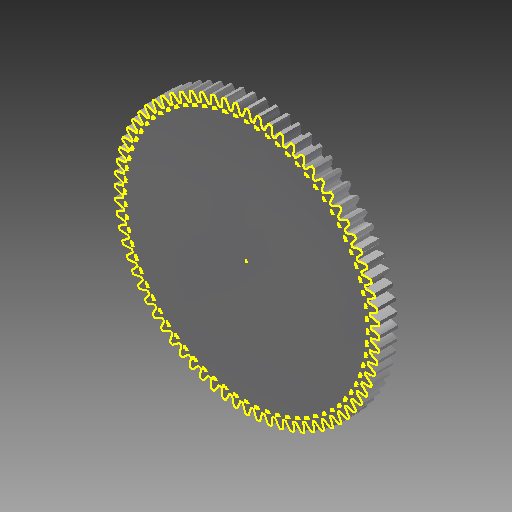
# Autodesk Inventor part: Цилиндрическое зубчатое зацепление2
Saved by Autodesk Inventor 2019 (Build 230136000, 136)
## iProperties
Created: 2020-02-27
Part Number: Цилиндрическое зубчатое зацепление2
Material: Steel
Document SubType Name: Modeling
Designer: Петров Иван
Categories: <?xml version="1.0" encoding="UTF-16"?> <MemberInstance><Categories><FamilyTemplate><FamilyTemplateParameter ValueType="xs:double" Id="1" ObjectReferenceKey="da_z" ObjectType="kUserParameterObject"/><FamilyTemplateParameter ValueType="xs:double" Id="2" ObjectReferenceKey="da_b" ObjectType="kUserParameterObject"/><FamilyTemplateParameter ValueType="xs:double" Id="3" ObjectReferenceKey="da_beta" ObjectType="kUserParameterObject"/><FamilyTemplateParameter ValueType="xs:double" Id="4" ObjectReferenceKey="da_da" ObjectType="kUserParameterObject"/><FamilyTemplateParameter ValueType="xs:double" Id="5" ObjectReferenceKey="da_aw" ObjectType="kUserParameterObject"/><FamilyTemplateParameter ValueType="xs:string" Id="6" ObjectReferenceKey="EAIAABAAAACIAQAAAAAAAIAAAAAAAAAA" ObjectType="83910656" SubObjectId="SurfaceGeometry"/></FamilyTemplate><ParamToTemplateMap><ParamToTemplate CategoryParameter="//CategoryParameter[@InternalName='046C89C9-8512-4d59-83FE-43B91F4F132A']" TemplateParameter="1"/><ParamToTemplate CategoryParameter="//CategoryParameter[@InternalName='2552DF32-E462-4b46-AEBF-C6C7768E72AC']" TemplateParameter="2"/><ParamToTemplate CategoryParameter="//CategoryParameter[@InternalName='C9EE641D-15FC-4fae-A226-E94C4372FDD7']" TemplateParameter="3"/><ParamToTemplate><ParamToTemplate CategoryParameter="//CategoryParameter[@InternalName='00B6519A-459B-49c7-AD84-2E56D39A5744']" ConstantValue="-1.297544"/></ParamToTemplate><ParamToTemplate><ParamToTemplate CategoryParameter="//CategoryParameter[@InternalName='04B31F0E-C7A6-4894-AA32-9629BEFACF47']" ConstantValue="1.000000"/></ParamToTemplate><ParamToTemplate><ParamToTemplate CategoryParameter="//CategoryParameter[@InternalName='43CBEC2E-7847-49e7-A936-2F7889FCB2D9']" ConstantValue="0.250000"/></ParamToTemplate><ParamToTemplate><ParamToTemplate CategoryParameter="//CategoryParameter[@InternalName='B1EFC894-105D-4ebd-86BF-FA20ED196853']" ConstantValue="0.350000"/></ParamToTemplate><ParamToTemplate><ParamToTemplate CategoryParameter="//CategoryParameter[@InternalName='51175063-3D10-4879-93E8-6246FE8B403D']" ConstantValue="2060000000.000000"/></ParamToTemplate><ParamToTemplate><ParamToTemplate CategoryParameter="//CategoryParameter[@InternalName='A3A52E27-4454-46a9-B0BD-C932399B70AF']" ConstantValue="0.300000"/></ParamToTemplate><ParamToTemplate><ParamToTemplate CategoryParameter="//CategoryParameter[@InternalName='91B76062-C214-41d9-B1B9-14D2AB99603D']" ConstantValue="0.137500"/></ParamToTemplate><ParamToTemplate><ParamToTemplate CategoryParameter="//CategoryParameter[@InternalName='374E806E-8B8A-4dda-A9AA-1039D6500AD2']" ConstantValue="7.272727"/></ParamToTemplate><ParamToTemplate><ParamToTemplate CategoryParameter="//CategoryParameter[@InternalName='2D373A89-B862-43d6-8D0B-0CBF12AB9F6C']" ConstantValue="0.523599"/></ParamToTemplate><ParamToTemplate CategoryParameter="//CategoryParameter[@InternalName='37777632-D6A2-4fac-9D53-DB8ACD95C989']" TemplateParameter="4"/><ParamToTemplate CategoryParameter="//CategoryParameter[@InternalName='FD1017F1-B727-4f7e-9707-0F86F1FF9423']" TemplateParameter="5"/><ParamToTemplate><ParamToTemplate CategoryParameter="//CategoryParameter[@InternalName='9E1B4470-B2D3-4ff1-B813-535BB4CDF51A']" ConstantValue="3520000.000000"/></ParamToTemplate><ParamToTemplate><ParamToTemplate CategoryParameter="//CategoryParameter[@InternalName='F8452263-BFF6-458c-9FB1-07C4B99E95CD']" ConstantValue="11400000.000000"/></ParamToTemplate><ParamToTemplate><ParamToTemplate CategoryParameter="//CategoryParameter[@InternalName='3E3BB259-FD49-497f-8171-6EBC954A3479']" ConstantValue="2.000000"/></ParamToTemplate><ParamToTemplate CategoryParameter="//CategoryParameter[@InternalName='27C3BAF2-7550-4e4b-AE2C-0DB134B7D9B7']" TemplateParameter="6"/></ParamToTemplateMap><Category DisplayName="Gear" InternalName="DC85795E-93AB-48d5-8EEE-5A27447B64BD" Mnemonic="Gear"><CategoryParameter DisplayName="z" InternalName="046C89C9-8512-4d59-83FE-43B91F4F132A" Mnemonic="z"/><CategoryParameter DisplayName="b" InternalName="2552DF32-E462-4b46-AEBF-C6C7768E72AC" Mnemonic="b"/><CategoryParameter DisplayName="||b|" InternalName="C9EE641D-15FC-4fae-A226-E94C4372FDD7" Mnemonic="beta"/><CategoryParameter DisplayName="x" InternalName="00B6519A-459B-49c7-AD84-2E56D39A5744" Mnemonic="x"/><CategoryParameter DisplayName="a*" InternalName="04B31F0E-C7A6-4894-AA32-9629BEFACF47" Mnemonic="a"/><CategoryParameter DisplayName="c*" InternalName="43CBEC2E-7847-49e7-A936-2F7889FCB2D9" Mnemonic="c"/><CategoryParameter DisplayName="r|.f|*" InternalName="B1EFC894-105D-4ebd-86BF-FA20ED196853" Mnemonic="rf"/><CategoryParameter DisplayName="E" InternalName="51175063-3D10-4879-93E8-6246FE8B403D" Mnemonic="E"/><CategoryParameter DisplayName="||m|" InternalName="A3A52E27-4454-46a9-B0BD-C932399B70AF" Mnemonic="mi"/><Category DisplayName="SpurGear" InternalName="26C5A22E-A91E-4dfd-A3B3-23CCAFAE1764" Mnemonic="SpurGear"><CategoryParameter DisplayName="m" InternalName="91B76062-C214-41d9-B1B9-14D2AB99603D" Mnemonic="m"/><CategoryParameter DisplayName="P" InternalName="374E806E-8B8A-4dda-A9AA-1039D6500AD2" Mnemonic="PP"/><CategoryParameter DisplayName="||a|" InternalName="2D373A89-B862-43d6-8D0B-0CBF12AB9F6C" Mnemonic="alpha"/><CategoryParameter DisplayName="d|.a|" InternalName="37777632-D6A2-4fac-9D53-DB8ACD95C989" Mnemonic="da"/><CategoryParameter DisplayName="a|.w|" InternalName="FD1017F1-B727-4f7e-9707-0F86F1FF9423" Mnemonic="aw"/><CategoryParameter DisplayName="||s||.Flim|" InternalName="9E1B4470-B2D3-4ff1-B813-535BB4CDF51A" Mnemonic="sFlim"/><CategoryParameter DisplayName="||s||.Hlim|" InternalName="F8452263-BFF6-458c-9FB1-07C4B99E95CD" Mnemonic="sHlim"/><CategoryParameter DisplayName="тип" InternalName="3E3BB259-FD49-497f-8171-6EBC954A3479" Mnemonic="type"/><CategoryParameter DisplayName="PitchDiameter" InternalName="27C3BAF2-7550-4e4b-AE2C-0DB134B7D9B7" Mnemonic="IDS_PITCHDIAM"/></Category></Category></Categories></MemberInstance>
Density: 1 g/cm^3
Appearance: Steel
CustomPartVersion: 1
Author: Петров Иван
Autodesk Inventor part; units mm, degrees
sketch "Sketch1" plane through (0, 0, 0) normal (0, 0, 1) x (1, 0, 0)
  circle A0 centre (0, 0) radius 49
  dimension "d0" = 98
  constraints: 1 centre point
  measures "d0" diameter of A0
extrude "Extrusion1" add sketch "Sketch1" along normal blind 7
ref_plane "Work Plane2" through (0, 0, 3.5) normal (0, 0, 1) x (1, 0, 0)
sketch "Sketch2" plane through (0, 0, 0) normal (0, 0, -1) x (-1, 0, 0)
  circle A0 centre (0, 0) radius 49 projected
  circle A1 centre (0, 0) radius 48
  dimension "d3" = 96
  constraints: 1 centre point, 1 coincident
  measures "d3" diameter of A1
surface extrude "Средний диаметр" sketch "Sketch2" against normal through all shown no curves A1
ref_plane "Work Plane8" through (0, 0, 0) normal (0.9990482, 0.0436194, 0) x (0, 0, 1)
ref_plane "Work Plane9" through (0, 0, 0) normal (1, 0, 0) x (0, 1, 0)
spur gear teeth "Цилиндрическое зубчатое зацепление" teeth 72 pitch diameter 99 tip diameter 98 root diameter 91.9943 face width 7 start plane through (0, 0, 0) normal (0, 0, -1) x (-1, 0, 0)
sketch "Эскиз3" plane through (0, 0, 7) normal (0, 0, 1) x (1, 0, 0)
  arc A0 (4.8028, -48.7641) -> (5.506, -45.6664) centre (-12.0114, -43.3185) ccw projected
  arc A1 (5.506, -45.6664) -> (6.5009, -45.5354) centre (0, 0) ccw projected
  arc A2 (6.5009, -45.5354) -> (7.9819, -48.3455) centre (22.8137, -38.7337) ccw projected
  arc A3 (7.9819, -48.3455) -> (9.0346, -48.1599) centre (0, 0) ccw projected
  arc A4 (9.0346, -48.1599) -> (9.4652, -45.0127) centre (-8.1902, -44.2005) ccw projected
  arc A5 (9.4652, -45.0127) -> (10.4449, -44.7955) centre (0, 0) ccw projected
  arc A6 (10.4449, -44.7955) -> (12.1651, -47.4659) centre (26.1028, -36.598) ccw projected
  arc A7 (12.1651, -47.4659) -> (13.1977, -47.1892) centre (0, 0) ccw projected
  arc A8 (13.1977, -47.1892) -> (13.3523, -44.0165) centre (-4.3067, -44.7461) ccw projected
  arc A9 (13.3523, -44.0165) -> (14.3093, -43.7148) centre (0, 0) ccw projected
  arc A10 (14.3093, -43.7148) -> (16.2557, -46.225) centre (29.1932, -34.1837) ccw projected
  arc A11 (16.2557, -46.225) -> (17.2603, -45.8594) centre (0, 0) ccw projected
  arc A12 (17.2603, -45.8594) -> (17.1377, -42.6853) centre (-0.3904, -44.9512) ccw projected
  arc A13 (17.1377, -42.6853) -> (18.0648, -42.3013) centre (0, 0) ccw projected
  arc A14 (18.0648, -42.3013) -> (20.2226, -44.6323) centre (32.0614, -31.5092) ccw projected
  arc A15 (20.2226, -44.6323) -> (21.1915, -44.1806) centre (0, 0) ccw projected
  arc A16 (21.1915, -44.1806) -> (20.7928, -41.0292) centre (3.5288, -44.8142) ccw projected
  arc A17 (20.7928, -41.0292) -> (21.6829, -40.5658) centre (0, 0) ccw projected
  arc A18 (21.6829, -40.5658) -> (24.0357, -42.7) centre (34.6856, -28.595) ccw projected
  arc A19 (24.0357, -42.7) -> (24.9614, -42.1655) centre (0, 0) ccw projected
  arc A20 (24.9614, -42.1655) -> (24.2896, -39.0609) centre (7.4212, -44.3361) ccw projected
  arc A21 (24.2896, -39.0609) -> (25.1359, -38.5217) centre (0, 0) ccw projected
  arc A22 (25.1359, -38.5217) -> (27.6657, -40.4426) centre (37.0458, -25.4632) ccw projected
  arc A23 (27.6657, -40.4426) -> (28.5414, -39.8295) centre (0, 0) ccw projected
  arc A24 (28.5414, -39.8295) -> (27.6016, -36.7952) centre (11.2571, -43.5206) ccw projected
  arc A25 (27.6016, -36.7952) -> (28.3977, -36.1844) centre (0, 0) ccw projected
  arc A26 (28.3977, -36.1844) -> (31.0853, -37.8775) centre (39.1241, -22.1375) ccw projected
  arc A27 (31.0853, -37.8775) -> (31.9042, -37.1904) centre (0, 0) ccw projected
  arc A28 (31.9042, -37.1904) -> (30.7034, -34.2496) centre (15.0073, -42.3739) ccw projected
  arc A29 (30.7034, -34.2496) -> (31.4433, -33.5717) centre (0, 0) ccw projected
  arc A30 (31.4433, -33.5717) -> (34.2682, -35.0241) centre (40.9046, -18.6434) ccw projected
  arc A31 (34.2682, -35.0241) -> (35.0241, -34.2682) centre (0, 0) ccw projected
  arc A32 (35.0241, -34.2682) -> (33.5717, -31.4433) centre (18.6434, -40.9046) ccw projected
  arc A33 (33.5717, -31.4433) -> (34.2496, -30.7034) centre (0, 0) ccw projected
  arc A34 (34.2496, -30.7034) -> (37.1904, -31.9042) centre (42.3739, -15.0073) ccw projected
  arc A35 (37.1904, -31.9042) -> (37.8775, -31.0853) centre (0, 0) ccw projected
  arc A36 (37.8775, -31.0853) -> (36.1844, -28.3977) centre (22.1375, -39.1241) ccw projected
  arc A37 (36.1844, -28.3977) -> (36.7952, -27.6016) centre (0, 0) ccw projected
  arc A38 (36.7952, -27.6016) -> (39.8295, -28.5414) centre (43.5206, -11.2571) ccw projected
  arc A39 (39.8295, -28.5414) -> (40.4426, -27.6657) centre (0, 0) ccw projected
  arc A40 (40.4426, -27.6657) -> (38.5217, -25.1359) centre (25.4632, -37.0458) ccw projected
  arc A41 (38.5217, -25.1359) -> (39.0609, -24.2896) centre (0, 0) ccw projected
  arc A42 (39.0609, -24.2896) -> (42.1655, -24.9614) centre (44.3361, -7.4212) ccw projected
  arc A43 (42.1655, -24.9614) -> (42.7, -24.0357) centre (0, 0) ccw projected
  arc A44 (42.7, -24.0357) -> (40.5658, -21.6829) centre (28.595, -34.6856) ccw projected
  arc A45 (40.5658, -21.6829) -> (41.0292, -20.7928) centre (0, 0) ccw projected
  arc A46 (41.0292, -20.7928) -> (44.1806, -21.1915) centre (44.8142, -3.5288) ccw projected
  arc A47 (44.1806, -21.1915) -> (44.6323, -20.2226) centre (0, 0) ccw projected
  arc A48 (44.6323, -20.2226) -> (42.3013, -18.0648) centre (31.5092, -32.0614) ccw projected
  arc A49 (42.3013, -18.0648) -> (42.6853, -17.1377) centre (0, 0) ccw projected
  arc A50 (42.6853, -17.1377) -> (45.8594, -17.2603) centre (44.9512, 0.3904) ccw projected
  arc A51 (45.8594, -17.2603) -> (46.225, -16.2557) centre (0, 0) ccw projected
  arc A52 (46.225, -16.2557) -> (43.7148, -14.3093) centre (34.1837, -29.1932) ccw projected
  arc A53 (43.7148, -14.3093) -> (44.0165, -13.3523) centre (0, 0) ccw projected
  arc A54 (44.0165, -13.3523) -> (47.1892, -13.1977) centre (44.7461, 4.3067) ccw projected
  arc A55 (47.1892, -13.1977) -> (47.4659, -12.1651) centre (0, 0) ccw projected
  arc A56 (47.4659, -12.1651) -> (44.7955, -10.4449) centre (36.598, -26.1028) ccw projected
  arc A57 (44.7955, -10.4449) -> (45.0127, -9.4652) centre (0, 0) ccw projected
  arc A58 (45.0127, -9.4652) -> (48.1599, -9.0346) centre (44.2005, 8.1902) ccw projected
  arc A59 (48.1599, -9.0346) -> (48.3455, -7.9819) centre (0, 0) ccw projected
  arc A60 (48.3455, -7.9819) -> (45.5354, -6.5009) centre (38.7337, -22.8137) ccw projected
  arc A61 (45.5354, -6.5009) -> (45.6664, -5.506) centre (0, 0) ccw projected
  arc A62 (45.6664, -5.506) -> (48.7641, -4.8028) centre (43.3185, 12.0114) ccw projected
  arc A63 (48.7641, -4.8028) -> (48.8572, -3.7379) centre (0, 0) ccw projected
  arc A64 (48.8572, -3.7379) -> (45.9287, -2.5075) centre (40.5746, -19.3511) ccw projected
  arc A65 (45.9287, -2.5075) -> (45.9725, -1.505) centre (0, 0) ccw projected
  arc A66 (45.9725, -1.505) -> (48.9971, -0.5345) centre (42.1068, 15.7411) ccw projected
  arc A67 (48.9971, -0.5345) -> (48.9971, 0.5345) centre (0, 0) ccw projected
  arc A68 (48.9971, 0.5345) -> (45.9725, 1.505) centre (42.1068, -15.7411) ccw projected
  arc A69 (45.9725, 1.505) -> (45.9287, 2.5075) centre (0, 0) ccw projected
  arc A70 (45.9287, 2.5075) -> (48.8572, 3.7379) centre (40.5746, 19.3511) ccw projected
  arc A71 (48.8572, 3.7379) -> (48.7641, 4.8028) centre (0, 0) ccw projected
  arc A72 (48.7641, 4.8028) -> (45.6664, 5.506) centre (43.3185, -12.0114) ccw projected
  arc A73 (45.6664, 5.506) -> (45.5354, 6.5009) centre (0, 0) ccw projected
  arc A74 (45.5354, 6.5009) -> (48.3455, 7.9819) centre (38.7337, 22.8137) ccw projected
  arc A75 (48.3455, 7.9819) -> (48.1599, 9.0346) centre (0, 0) ccw projected
  arc A76 (48.1599, 9.0346) -> (45.0127, 9.4652) centre (44.2005, -8.1902) ccw projected
  arc A77 (45.0127, 9.4652) -> (44.7955, 10.4449) centre (0, 0) ccw projected
  arc A78 (44.7955, 10.4449) -> (47.4659, 12.1651) centre (36.598, 26.1028) ccw projected
  arc A79 (47.4659, 12.1651) -> (47.1892, 13.1977) centre (0, 0) ccw projected
  arc A80 (47.1892, 13.1977) -> (44.0165, 13.3523) centre (44.7461, -4.3067) ccw projected
  arc A81 (44.0165, 13.3523) -> (43.7148, 14.3093) centre (0, 0) ccw projected
  arc A82 (43.7148, 14.3093) -> (46.225, 16.2557) centre (34.1837, 29.1932) ccw projected
  arc A83 (46.225, 16.2557) -> (45.8594, 17.2603) centre (0, 0) ccw projected
  arc A84 (45.8594, 17.2603) -> (42.6853, 17.1377) centre (44.9512, -0.3904) ccw projected
  arc A85 (42.6853, 17.1377) -> (42.3013, 18.0648) centre (0, 0) ccw projected
  arc A86 (42.3013, 18.0648) -> (44.6323, 20.2226) centre (31.5092, 32.0614) ccw projected
  arc A87 (44.6323, 20.2226) -> (44.1806, 21.1915) centre (0, 0) ccw projected
  arc A88 (44.1806, 21.1915) -> (41.0292, 20.7928) centre (44.8142, 3.5288) ccw projected
  arc A89 (41.0292, 20.7928) -> (40.5658, 21.6829) centre (0, 0) ccw projected
  arc A90 (40.5658, 21.6829) -> (42.7, 24.0357) centre (28.595, 34.6856) ccw projected
  arc A91 (42.7, 24.0357) -> (42.1655, 24.9614) centre (0, 0) ccw projected
  arc A92 (42.1655, 24.9614) -> (39.0609, 24.2896) centre (44.3361, 7.4212) ccw projected
  arc A93 (39.0609, 24.2896) -> (38.5217, 25.1359) centre (0, 0) ccw projected
  arc A94 (38.5217, 25.1359) -> (40.4426, 27.6657) centre (25.4632, 37.0458) ccw projected
  arc A95 (40.4426, 27.6657) -> (39.8295, 28.5414) centre (0, 0) ccw projected
  arc A96 (39.8295, 28.5414) -> (36.7952, 27.6016) centre (43.5206, 11.2571) ccw projected
  arc A97 (36.7952, 27.6016) -> (36.1844, 28.3977) centre (0, 0) ccw projected
  arc A98 (36.1844, 28.3977) -> (37.8775, 31.0853) centre (22.1375, 39.1241) ccw projected
  arc A99 (37.8775, 31.0853) -> (37.1904, 31.9042) centre (0, 0) ccw projected
  arc A100 (37.1904, 31.9042) -> (34.2496, 30.7034) centre (42.3739, 15.0073) ccw projected
  arc A101 (34.2496, 30.7034) -> (33.5717, 31.4433) centre (0, 0) ccw projected
  arc A102 (33.5717, 31.4433) -> (35.0241, 34.2682) centre (18.6434, 40.9046) ccw projected
  arc A103 (35.0241, 34.2682) -> (34.2682, 35.0241) centre (0, 0) ccw projected
  arc A104 (34.2682, 35.0241) -> (31.4433, 33.5717) centre (40.9046, 18.6434) ccw projected
  arc A105 (31.4433, 33.5717) -> (30.7034, 34.2496) centre (0, 0) ccw projected
  arc A106 (30.7034, 34.2496) -> (31.9042, 37.1904) centre (15.0073, 42.3739) ccw projected
  arc A107 (31.9042, 37.1904) -> (31.0853, 37.8775) centre (0, 0) ccw projected
  arc A108 (31.0853, 37.8775) -> (28.3977, 36.1844) centre (39.1241, 22.1375) ccw projected
  arc A109 (28.3977, 36.1844) -> (27.6016, 36.7952) centre (0, 0) ccw projected
  arc A110 (27.6016, 36.7952) -> (28.5414, 39.8295) centre (11.2571, 43.5206) ccw projected
  arc A111 (28.5414, 39.8295) -> (27.6657, 40.4426) centre (0, 0) ccw projected
  arc A112 (27.6657, 40.4426) -> (25.1359, 38.5217) centre (37.0458, 25.4632) ccw projected
  arc A113 (25.1359, 38.5217) -> (24.2896, 39.0609) centre (0, 0) ccw projected
  arc A114 (24.2896, 39.0609) -> (24.9614, 42.1655) centre (7.4212, 44.3361) ccw projected
  arc A115 (24.9614, 42.1655) -> (24.0357, 42.7) centre (0, 0) ccw projected
  arc A116 (24.0357, 42.7) -> (21.6829, 40.5658) centre (34.6856, 28.595) ccw projected
  arc A117 (21.6829, 40.5658) -> (20.7928, 41.0292) centre (0, 0) ccw projected
  arc A118 (20.7928, 41.0292) -> (21.1915, 44.1806) centre (3.5288, 44.8142) ccw projected
  arc A119 (21.1915, 44.1806) -> (20.2226, 44.6323) centre (0, 0) ccw projected
  arc A120 (20.2226, 44.6323) -> (18.0648, 42.3013) centre (32.0614, 31.5092) ccw projected
  arc A121 (18.0648, 42.3013) -> (17.1377, 42.6853) centre (0, 0) ccw projected
  arc A122 (17.1377, 42.6853) -> (17.2603, 45.8594) centre (-0.3904, 44.9512) ccw projected
  arc A123 (17.2603, 45.8594) -> (16.2557, 46.225) centre (0, 0) ccw projected
  arc A124 (16.2557, 46.225) -> (14.3093, 43.7148) centre (29.1932, 34.1837) ccw projected
  arc A125 (14.3093, 43.7148) -> (13.3523, 44.0165) centre (0, 0) ccw projected
  arc A126 (13.3523, 44.0165) -> (13.1977, 47.1892) centre (-4.3067, 44.7461) ccw projected
  arc A127 (13.1977, 47.1892) -> (12.1651, 47.4659) centre (0, 0) ccw projected
  arc A128 (12.1651, 47.4659) -> (10.4449, 44.7955) centre (26.1028, 36.598) ccw projected
  arc A129 (10.4449, 44.7955) -> (9.4652, 45.0127) centre (0, 0) ccw projected
  arc A130 (9.4652, 45.0127) -> (9.0346, 48.1599) centre (-8.1902, 44.2005) ccw projected
  arc A131 (9.0346, 48.1599) -> (7.9819, 48.3455) centre (0, 0) ccw projected
  arc A132 (7.9819, 48.3455) -> (6.5009, 45.5354) centre (22.8137, 38.7337) ccw projected
  arc A133 (6.5009, 45.5354) -> (5.506, 45.6664) centre (0, 0) ccw projected
  arc A134 (5.506, 45.6664) -> (4.8028, 48.7641) centre (-12.0114, 43.3185) ccw projected
  arc A135 (4.8028, 48.7641) -> (3.7379, 48.8572) centre (0, 0) ccw projected
  arc A136 (3.7379, 48.8572) -> (2.5075, 45.9287) centre (19.3511, 40.5746) ccw projected
  arc A137 (2.5075, 45.9287) -> (1.505, 45.9725) centre (0, 0) ccw projected
  arc A138 (1.505, 45.9725) -> (0.5345, 48.9971) centre (-15.7411, 42.1068) ccw projected
  arc A139 (0.5345, 48.9971) -> (-0.5345, 48.9971) centre (0, 0) ccw projected
  arc A140 (-0.5345, 48.9971) -> (-1.505, 45.9725) centre (15.7411, 42.1068) ccw projected
  arc A141 (-1.505, 45.9725) -> (-2.5075, 45.9287) centre (0, 0) ccw projected
  arc A142 (-2.5075, 45.9287) -> (-3.7379, 48.8572) centre (-19.3511, 40.5746) ccw projected
  arc A143 (3.7379, -48.8572) -> (4.8028, -48.7641) centre (0, 0) ccw projected
  arc A144 (-4.8028, 48.7641) -> (-5.506, 45.6664) centre (12.0114, 43.3185) ccw projected
  arc A145 (-5.506, 45.6664) -> (-6.5009, 45.5354) centre (0, 0) ccw projected
  arc A146 (-6.5009, 45.5354) -> (-7.9819, 48.3455) centre (-22.8137, 38.7337) ccw projected
  arc A147 (-7.9819, 48.3455) -> (-9.0346, 48.1599) centre (0, 0) ccw projected
  arc A148 (-9.0346, 48.1599) -> (-9.4652, 45.0127) centre (8.1902, 44.2005) ccw projected
  arc A149 (-9.4652, 45.0127) -> (-10.4449, 44.7955) centre (0, 0) ccw projected
  arc A150 (-10.4449, 44.7955) -> (-12.1651, 47.4659) centre (-26.1028, 36.598) ccw projected
  arc A151 (-12.1651, 47.4659) -> (-13.1977, 47.1892) centre (0, 0) ccw projected
  arc A152 (-13.1977, 47.1892) -> (-13.3523, 44.0165) centre (4.3067, 44.7461) ccw projected
  arc A153 (-13.3523, 44.0165) -> (-14.3093, 43.7148) centre (0, 0) ccw projected
  arc A154 (-14.3093, 43.7148) -> (-16.2557, 46.225) centre (-29.1932, 34.1837) ccw projected
  arc A155 (-16.2557, 46.225) -> (-17.2603, 45.8594) centre (0, 0) ccw projected
  arc A156 (-17.2603, 45.8594) -> (-17.1377, 42.6853) centre (0.3904, 44.9512) ccw projected
  arc A157 (-17.1377, 42.6853) -> (-18.0648, 42.3013) centre (0, 0) ccw projected
  arc A158 (-18.0648, 42.3013) -> (-20.2226, 44.6323) centre (-32.0614, 31.5092) ccw projected
  arc A159 (-20.2226, 44.6323) -> (-21.1915, 44.1806) centre (0, 0) ccw projected
  arc A160 (-21.1915, 44.1806) -> (-20.7928, 41.0292) centre (-3.5288, 44.8142) ccw projected
  arc A161 (-20.7928, 41.0292) -> (-21.6829, 40.5658) centre (0, 0) ccw projected
  arc A162 (-21.6829, 40.5658) -> (-24.0357, 42.7) centre (-34.6856, 28.595) ccw projected
  arc A163 (-24.0357, 42.7) -> (-24.9614, 42.1655) centre (0, 0) ccw projected
  arc A164 (-24.9614, 42.1655) -> (-24.2896, 39.0609) centre (-7.4212, 44.3361) ccw projected
  arc A165 (-24.2896, 39.0609) -> (-25.1359, 38.5217) centre (0, 0) ccw projected
  arc A166 (-25.1359, 38.5217) -> (-27.6657, 40.4426) centre (-37.0458, 25.4632) ccw projected
  arc A167 (-27.6657, 40.4426) -> (-28.5414, 39.8295) centre (0, 0) ccw projected
  arc A168 (-28.5414, 39.8295) -> (-27.6016, 36.7952) centre (-11.2571, 43.5206) ccw projected
  arc A169 (-27.6016, 36.7952) -> (-28.3977, 36.1844) centre (0, 0) ccw projected
  arc A170 (-28.3977, 36.1844) -> (-31.0853, 37.8775) centre (-39.1241, 22.1375) ccw projected
  arc A171 (-31.0853, 37.8775) -> (-31.9042, 37.1904) centre (0, 0) ccw projected
  arc A172 (-31.9042, 37.1904) -> (-30.7034, 34.2496) centre (-15.0073, 42.3739) ccw projected
  arc A173 (-30.7034, 34.2496) -> (-31.4433, 33.5717) centre (0, 0) ccw projected
  arc A174 (-31.4433, 33.5717) -> (-34.2682, 35.0241) centre (-40.9046, 18.6434) ccw projected
  arc A175 (-34.2682, 35.0241) -> (-35.0241, 34.2682) centre (0, 0) ccw projected
  arc A176 (-35.0241, 34.2682) -> (-33.5717, 31.4433) centre (-18.6434, 40.9046) ccw projected
  arc A177 (-33.5717, 31.4433) -> (-34.2496, 30.7034) centre (0, 0) ccw projected
  arc A178 (-34.2496, 30.7034) -> (-37.1904, 31.9042) centre (-42.3739, 15.0073) ccw projected
  arc A179 (-37.1904, 31.9042) -> (-37.8775, 31.0853) centre (0, 0) ccw projected
  arc A180 (-37.8775, 31.0853) -> (-36.1844, 28.3977) centre (-22.1375, 39.1241) ccw projected
  arc A181 (-36.1844, 28.3977) -> (-36.7952, 27.6016) centre (0, 0) ccw projected
  arc A182 (-36.7952, 27.6016) -> (-39.8295, 28.5414) centre (-43.5206, 11.2571) ccw projected
  arc A183 (-39.8295, 28.5414) -> (-40.4426, 27.6657) centre (0, 0) ccw projected
  arc A184 (-40.4426, 27.6657) -> (-38.5217, 25.1359) centre (-25.4632, 37.0458) ccw projected
  arc A185 (-38.5217, 25.1359) -> (-39.0609, 24.2896) centre (0, 0) ccw projected
  arc A186 (-39.0609, 24.2896) -> (-42.1655, 24.9614) centre (-44.3361, 7.4212) ccw projected
  arc A187 (-42.1655, 24.9614) -> (-42.7, 24.0357) centre (0, 0) ccw projected
  arc A188 (-42.7, 24.0357) -> (-40.5658, 21.6829) centre (-28.595, 34.6856) ccw projected
  arc A189 (-40.5658, 21.6829) -> (-41.0292, 20.7928) centre (0, 0) ccw projected
  arc A190 (-41.0292, 20.7928) -> (-44.1806, 21.1915) centre (-44.8142, 3.5288) ccw projected
  arc A191 (-44.1806, 21.1915) -> (-44.6323, 20.2226) centre (0, 0) ccw projected
  arc A192 (-44.6323, 20.2226) -> (-42.3013, 18.0648) centre (-31.5092, 32.0614) ccw projected
  arc A193 (-42.3013, 18.0648) -> (-42.6853, 17.1377) centre (0, 0) ccw projected
  arc A194 (-42.6853, 17.1377) -> (-45.8594, 17.2603) centre (-44.9512, -0.3904) ccw projected
  arc A195 (-45.8594, 17.2603) -> (-46.225, 16.2557) centre (0, 0) ccw projected
  arc A196 (-46.225, 16.2557) -> (-43.7148, 14.3093) centre (-34.1837, 29.1932) ccw projected
  arc A197 (-43.7148, 14.3093) -> (-44.0165, 13.3523) centre (0, 0) ccw projected
  arc A198 (-44.0165, 13.3523) -> (-47.1892, 13.1977) centre (-44.7461, -4.3067) ccw projected
  arc A199 (-47.1892, 13.1977) -> (-47.4659, 12.1651) centre (0, 0) ccw projected
  arc A200 (-47.4659, 12.1651) -> (-44.7955, 10.4449) centre (-36.598, 26.1028) ccw projected
  arc A201 (-44.7955, 10.4449) -> (-45.0127, 9.4652) centre (0, 0) ccw projected
  arc A202 (-45.0127, 9.4652) -> (-48.1599, 9.0346) centre (-44.2005, -8.1902) ccw projected
  arc A203 (-48.1599, 9.0346) -> (-48.3455, 7.9819) centre (0, 0) ccw projected
  arc A204 (-48.3455, 7.9819) -> (-45.5354, 6.5009) centre (-38.7337, 22.8137) ccw projected
  arc A205 (-45.5354, 6.5009) -> (-45.6664, 5.506) centre (0, 0) ccw projected
  arc A206 (-45.6664, 5.506) -> (-48.7641, 4.8028) centre (-43.3185, -12.0114) ccw projected
  arc A207 (-48.7641, 4.8028) -> (-48.8572, 3.7379) centre (0, 0) ccw projected
  arc A208 (-48.8572, 3.7379) -> (-45.9287, 2.5075) centre (-40.5746, 19.3511) ccw projected
  arc A209 (-45.9287, 2.5075) -> (-45.9725, 1.505) centre (0, 0) ccw projected
  arc A210 (-45.9725, 1.505) -> (-48.9971, 0.5345) centre (-42.1068, -15.7411) ccw projected
  arc A211 (-48.9971, 0.5345) -> (-48.9971, -0.5345) centre (0, 0) ccw projected
  arc A212 (-48.9971, -0.5345) -> (-45.9725, -1.505) centre (-42.1068, 15.7411) ccw projected
  arc A213 (-45.9725, -1.505) -> (-45.9287, -2.5075) centre (0, 0) ccw projected
  arc A214 (-45.9287, -2.5075) -> (-48.8572, -3.7379) centre (-40.5746, -19.3511) ccw projected
  arc A215 (-48.8572, -3.7379) -> (-48.7641, -4.8028) centre (0, 0) ccw projected
  arc A216 (-48.7641, -4.8028) -> (-45.6664, -5.506) centre (-43.3185, 12.0114) ccw projected
  arc A217 (-45.6664, -5.506) -> (-45.5354, -6.5009) centre (0, 0) ccw projected
  arc A218 (-45.5354, -6.5009) -> (-48.3455, -7.9819) centre (-38.7337, -22.8137) ccw projected
  arc A219 (-48.3455, -7.9819) -> (-48.1599, -9.0346) centre (0, 0) ccw projected
  arc A220 (-48.1599, -9.0346) -> (-45.0127, -9.4652) centre (-44.2005, 8.1902) ccw projected
  arc A221 (-45.0127, -9.4652) -> (-44.7955, -10.4449) centre (0, 0) ccw projected
  arc A222 (-44.7955, -10.4449) -> (-47.4659, -12.1651) centre (-36.598, -26.1028) ccw projected
  arc A223 (-47.4659, -12.1651) -> (-47.1892, -13.1977) centre (0, 0) ccw projected
  arc A224 (-47.1892, -13.1977) -> (-44.0165, -13.3523) centre (-44.7461, 4.3067) ccw projected
  arc A225 (-44.0165, -13.3523) -> (-43.7148, -14.3093) centre (0, 0) ccw projected
  arc A226 (-43.7148, -14.3093) -> (-46.225, -16.2557) centre (-34.1837, -29.1932) ccw projected
  arc A227 (-46.225, -16.2557) -> (-45.8594, -17.2603) centre (0, 0) ccw projected
  arc A228 (-45.8594, -17.2603) -> (-42.6853, -17.1377) centre (-44.9512, 0.3904) ccw projected
  arc A229 (-42.6853, -17.1377) -> (-42.3013, -18.0648) centre (0, 0) ccw projected
  arc A230 (-42.3013, -18.0648) -> (-44.6323, -20.2226) centre (-31.5092, -32.0614) ccw projected
  arc A231 (-44.6323, -20.2226) -> (-44.1806, -21.1915) centre (0, 0) ccw projected
  arc A232 (-44.1806, -21.1915) -> (-41.0292, -20.7928) centre (-44.8142, -3.5288) ccw projected
  arc A233 (-41.0292, -20.7928) -> (-40.5658, -21.6829) centre (0, 0) ccw projected
  arc A234 (-40.5658, -21.6829) -> (-42.7, -24.0357) centre (-28.595, -34.6856) ccw projected
  arc A235 (-42.7, -24.0357) -> (-42.1655, -24.9614) centre (0, 0) ccw projected
  arc A236 (-42.1655, -24.9614) -> (-39.0609, -24.2896) centre (-44.3361, -7.4212) ccw projected
  arc A237 (-39.0609, -24.2896) -> (-38.5217, -25.1359) centre (0, 0) ccw projected
  arc A238 (-38.5217, -25.1359) -> (-40.4426, -27.6657) centre (-25.4632, -37.0458) ccw projected
  arc A239 (-40.4426, -27.6657) -> (-39.8295, -28.5414) centre (0, 0) ccw projected
  arc A240 (-39.8295, -28.5414) -> (-36.7952, -27.6016) centre (-43.5206, -11.2571) ccw projected
  arc A241 (-36.7952, -27.6016) -> (-36.1844, -28.3977) centre (0, 0) ccw projected
  arc A242 (-36.1844, -28.3977) -> (-37.8775, -31.0853) centre (-22.1375, -39.1241) ccw projected
  arc A243 (-37.8775, -31.0853) -> (-37.1904, -31.9042) centre (0, 0) ccw projected
  arc A244 (-37.1904, -31.9042) -> (-34.2496, -30.7034) centre (-42.3739, -15.0073) ccw projected
  arc A245 (-34.2496, -30.7034) -> (-33.5717, -31.4433) centre (0, 0) ccw projected
  arc A246 (-33.5717, -31.4433) -> (-35.0241, -34.2682) centre (-18.6434, -40.9046) ccw projected
  arc A247 (-35.0241, -34.2682) -> (-34.2682, -35.0241) centre (0, 0) ccw projected
  arc A248 (-34.2682, -35.0241) -> (-31.4433, -33.5717) centre (-40.9046, -18.6434) ccw projected
  arc A249 (-31.4433, -33.5717) -> (-30.7034, -34.2496) centre (0, 0) ccw projected
  arc A250 (-30.7034, -34.2496) -> (-31.9042, -37.1904) centre (-15.0073, -42.3739) ccw projected
  arc A251 (-31.9042, -37.1904) -> (-31.0853, -37.8775) centre (0, 0) ccw projected
  arc A252 (-31.0853, -37.8775) -> (-28.3977, -36.1844) centre (-39.1241, -22.1375) ccw projected
  arc A253 (-28.3977, -36.1844) -> (-27.6016, -36.7952) centre (0, 0) ccw projected
  arc A254 (-27.6016, -36.7952) -> (-28.5414, -39.8295) centre (-11.2571, -43.5206) ccw projected
  arc A255 (-28.5414, -39.8295) -> (-27.6657, -40.4426) centre (0, 0) ccw projected
  arc A256 (-27.6657, -40.4426) -> (-25.1359, -38.5217) centre (-37.0458, -25.4632) ccw projected
  arc A257 (-25.1359, -38.5217) -> (-24.2896, -39.0609) centre (0, 0) ccw projected
  arc A258 (-24.2896, -39.0609) -> (-24.9614, -42.1655) centre (-7.4212, -44.3361) ccw projected
  arc A259 (-24.9614, -42.1655) -> (-24.0357, -42.7) centre (0, 0) ccw projected
  arc A260 (-24.0357, -42.7) -> (-21.6829, -40.5658) centre (-34.6856, -28.595) ccw projected
  arc A261 (-21.6829, -40.5658) -> (-20.7928, -41.0292) centre (0, 0) ccw projected
  arc A262 (-20.7928, -41.0292) -> (-21.1915, -44.1806) centre (-3.5288, -44.8142) ccw projected
  arc A263 (-21.1915, -44.1806) -> (-20.2226, -44.6323) centre (0, 0) ccw projected
  arc A264 (-20.2226, -44.6323) -> (-18.0648, -42.3013) centre (-32.0614, -31.5092) ccw projected
  arc A265 (-18.0648, -42.3013) -> (-17.1377, -42.6853) centre (0, 0) ccw projected
  arc A266 (-17.1377, -42.6853) -> (-17.2603, -45.8594) centre (0.3904, -44.9512) ccw projected
  arc A267 (-17.2603, -45.8594) -> (-16.2557, -46.225) centre (0, 0) ccw projected
  arc A268 (-16.2557, -46.225) -> (-14.3093, -43.7148) centre (-29.1932, -34.1837) ccw projected
  arc A269 (-14.3093, -43.7148) -> (-13.3523, -44.0165) centre (0, 0) ccw projected
  arc A270 (-13.3523, -44.0165) -> (-13.1977, -47.1892) centre (4.3067, -44.7461) ccw projected
  arc A271 (-13.1977, -47.1892) -> (-12.1651, -47.4659) centre (0, 0) ccw projected
  arc A272 (-12.1651, -47.4659) -> (-10.4449, -44.7955) centre (-26.1028, -36.598) ccw projected
  arc A273 (-10.4449, -44.7955) -> (-9.4652, -45.0127) centre (0, 0) ccw projected
  arc A274 (-9.4652, -45.0127) -> (-9.0346, -48.1599) centre (8.1902, -44.2005) ccw projected
  arc A275 (-9.0346, -48.1599) -> (-7.9819, -48.3455) centre (0, 0) ccw projected
  arc A276 (-7.9819, -48.3455) -> (-6.5009, -45.5354) centre (-22.8137, -38.7337) ccw projected
  arc A277 (-6.5009, -45.5354) -> (-5.506, -45.6664) centre (0, 0) ccw projected
  arc A278 (-5.506, -45.6664) -> (-4.8028, -48.7641) centre (12.0114, -43.3185) ccw projected
  arc A279 (-4.8028, -48.7641) -> (-3.7379, -48.8572) centre (0, 0) ccw projected
  arc A280 (-3.7379, -48.8572) -> (-2.5075, -45.9287) centre (-19.3511, -40.5746) ccw projected
  arc A281 (-2.5075, -45.9287) -> (-1.505, -45.9725) centre (0, 0) ccw projected
  arc A282 (-1.505, -45.9725) -> (-0.5345, -48.9971) centre (15.7411, -42.1068) ccw projected
  arc A283 (-0.5345, -48.9971) -> (0.5345, -48.9971) centre (0, 0) ccw projected
  arc A284 (0.5345, -48.9971) -> (1.505, -45.9725) centre (-15.7411, -42.1068) ccw projected
  arc A285 (1.505, -45.9725) -> (2.5075, -45.9287) centre (0, 0) ccw projected
  arc A286 (2.5075, -45.9287) -> (3.7379, -48.8572) centre (19.3511, -40.5746) ccw projected
  arc A287 (-3.7379, 48.8572) -> (-4.8028, 48.7641) centre (0, 0) ccw projected
equation "\"d0\" = da_da"
equation "\"d1\" = da_b"
equation "\"d3\" = da_dw"
equation "\"da_da\" = 98"
equation "\"da_b\" = 7"
equation "\"da_dw\" = 96"
body "Solid1"
body "Srf1"
